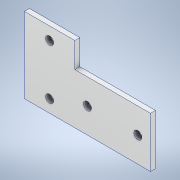
# Autodesk Inventor part: FrameJointL2020
Saved by Autodesk Inventor 2022.2 (Build 262287010, 287A)
## iProperties
Created: 2022-03-21
Part Number: FrameJointL2020
Material: アルミニウム 6061
Document SubType Name: Modeling
Designer: YusukeKunita
Density: 2.7 g/cm^3
Appearance: アルミニウム - フラット
Author: YusukeKunita
Autodesk Inventor part; units mm, degrees
ref_plane "YZ Plane" through (0, 0, 0) normal (1, 0, 0) x (0, 1, 0)
ref_plane "XZ Plane" through (0, 0, 0) normal (0, 1, 0) x (-1, 0, 0)
ref_plane "XY Plane" through (0, 0, 0) normal (0, 0, 1) x (1, 0, 0)
sketch "スケッチ1" plane through (0, 0, 0) normal (1, 0, 0) x (0, 1, 0)
  line L0 (0, 0) -> (50, 0)
  line L1 (50, 0) -> (50, 20)
  line L2 (50, 20) -> (0, 20)
  line L3 (0, 20) -> (0, 0)
  line L4 (0, 0) -> (20, 0)
  line L5 (20, 0) -> (20, 30)
  line L6 (20, 30) -> (0, 30)
  line L7 (0, 30) -> (0, 0)
  point P0 (0, 20)
  point P1 (20, 20)
  point P2 (20, 0)
  point P3 (20, 0)
  dimension "d0" = 20
  dimension "d1" = 20
  dimension "d2" = 30
  dimension "d3" = 30
  constraints: 16 end point, 4 parallel, 2 horizontal, 2 perpendicular
  measures "d0" distance of L0.end L1.end
  measures "d1" distance of L5.end L6.end
  measures "d2" distance between parallel lines of L5 L1
  measures "d3" distance of L4.end L5.end
extrude "押し出し1" add sketch "スケッチ1" along normal blind 2
sketch "スケッチ2" plane through (2, 0, 0) normal (1, 0, 0) x (0, 0, -1)
  line L0 (-30, 20) -> (-30, 0) projected
  line L1 (-30, 10) -> (0, 10) construction
  line L2 (0, 0) -> (0, 50) projected
  line L3 (0, 50) -> (-20, 50) projected
  line L4 (-10, 50) -> (-10, 0) construction
  line L5 (-30, 0) -> (0, 0) projected
  point P0 (-25, 10)
  point P1 (-5, 10)
  point P2 (-10, 25)
  point P3 (-10, 45)
  dimension "d6" = 20
  dimension "d7" = 5
  dimension "d8" = 20
  dimension "d9" = 5
  constraints: 5 point on line, 4 end point, 3 midpoint, 1 horizontal, 1 perpendicular
  measures "d6" distance of point (-10, 45) point (-10, 25)
  measures "d7" distance from line of L3 point (-10, 45)
  measures "d8" distance of point (-5, 10) point (-25, 10)
  measures "d9" distance from line of L0 point (-25, 10)
hole "穴1" at (2, 10, 25) at (2, 10, 5) at (2, 25, 10) at (2, 45, 10) direction (-1, 0, 0) diameter 3.2 end through all
